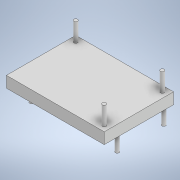
# Autodesk Inventor part: Divider_NodeMCU_Sipeed
Saved by Autodesk Inventor 2021 (Build 250183000, 183)
## iProperties
Created: 2023-10-10
Part Number: Divider_NodeMCU_Sipeed
Material: Generic
Document SubType Name: Modeling
Designer: 21seblin
Density: 1 g/cm^3
Appearance: Default
Author: 21seblin
Autodesk Inventor part; units mm, degrees
ref_plane "YZ Plane" through (0, 0, 0) normal (1, 0, 0) x (0, 1, 0)
ref_plane "XZ Plane" through (0, 0, 0) normal (0, 1, 0) x (-1, 0, 0)
ref_plane "XY Plane" through (0, 0, 0) normal (0, 0, 1) x (1, 0, 0)
sketch "Sketch1" plane through (0, 0, 0) normal (0, 1, 0) x (-1, 0, 0)
  line L0 (26.25, 18.6) -> (-26.25, 18.6)
  line L1 (-26.25, 18.6) -> (-26.25, -18.6)
  line L2 (-26.25, -18.6) -> (26.25, -18.6)
  line L3 (26.25, -18.6) -> (26.25, 18.6)
  line L4 (26.25, 18.6) -> (-26.25, -18.6) construction
  line L5 (-26.25, 18.6) -> (26.25, -18.6) construction
  line L6 (-26.25, -18.6) -> (-23.25, -18.6)
  point P0 (0, 0)
  dimension "d0" = 52.5
  dimension "d1" = 37.2
  dimension "d2" = 3
  constraints: 14 end point, 2 midpoint, 2 parallel, 1 horizontal, 1 perpendicular, 1 point on line
  measures "d0" distance of L1.end L2.end
  measures "d1" distance of L0.end L1.end
  measures "d2" distance of L6.end L1.end
extrude "Extrusion1" add sketch "Sketch1" along normal blind 6
sketch "Sketch2" plane through (0, 6, 0) normal (0, 1, 0) x (1, 0, 0)
  line L0 (26.25, 18.6) -> (-26.25, 18.6) projected
  line L1 (26.25, 18.6) -> (26.25, 15.6)
  line L2 (26.25, -18.6) -> (26.25, 18.6) projected
  line L3 (26.25, 18.6) -> (23.25, 18.6)
  line L4 (23.25, 18.6) -> (23.25, 15.6)
  circle A0 centre (23.25, 15.6) radius 1
  line L5 (26.25, 0) -> (18.0402, 0)
  line L6 (0, 18.6) -> (0, 10.2391)
  circle A1 centre (23.25, -15.6) radius 1
  circle A2 centre (-23.25, 15.6) radius 1
  point P0 (0, 0)
  dimension "d5" = 3
  dimension "d6" = 3
  dimension "d7" = 2
  constraints: 10 end point, 3 centre point, 2 midpoint, 2 point on line, 2 symmetric about line, 2 vertical, 1 coincident, 1 horizontal, 2 other
  measures "d5" distance of L0.start L1.end
  measures "d6" distance of L0.start L3.end
  measures "d7" diameter of A0
extrude "Extrusion2" add sketch "Sketch2" along normal blind 10
sketch "Sketch4" plane through (0, 0, 0) normal (0, -1, 0) x (1, 0, 0)
  line L0 (26.25, -18.6) -> (-26.25, -18.6) projected
  line L1 (-26.25, -18.6) -> (-26.25, -16.6)
  line L2 (-26.25, -18.6) -> (-26.25, 18.6) projected
  line L3 (-26.25, -16.6) -> (-23, -16.6)
  circle A0 centre (-23, -16.6) radius 1
  line L4 (-23, -16.6) -> (-23, 8.4)
  line L5 (-23, -4.1) -> (-16.8136, -4.1)
  circle A1 centre (-23, 8.4) radius 1
  line L6 (0, -18.6) -> (0, -14.1147)
  circle A2 centre (23, -16.6) radius 1
  circle A3 centre (23, 8.4) radius 1
  point P0 (0, 0)
  dimension "d16" = 2
  dimension "d17" = 3.25
  dimension "d18" = 2
  dimension "d19" = 25
  constraints: 10 end point, 4 centre point, 3 symmetric about line, 2 horizontal, 2 midpoint, 2 vertical, 1 coincident, 1 point on line, 3 other
  measures "d16" distance of L0.end L1.end
  measures "d17" distance of L1.end L3.end
  measures "d18" diameter of A0
  measures "d19" distance of L4.start L4.end
extrude "Extrusion4" add sketch "Sketch4" along normal blind 10
body "Solid1"
